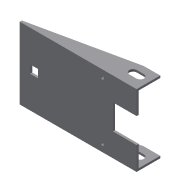
# Autodesk Inventor part: U-profil 100x40 - pod case
Saved by Autodesk Inventor 2015 (Build 190159000, 159)
## iProperties
Created: 2015-01-09
Part Number: U-profil 100x40 - pod case
Material: Všeobecné
Document SubType Name: Modeling
Designer: Michal
Density: 1 g/cm^3
Appearance: Výchozí
Author: Michal
Autodesk Inventor part; units mm, degrees
ref_plane "YZ Plane" through (0, 0, 0) normal (1, 0, 0) x (0, 1, 0)
ref_plane "XZ Plane" through (0, 0, 0) normal (0, 1, 0) x (-1, 0, 0)
ref_plane "XY Plane" through (0, 0, 0) normal (0, 0, 1) x (1, 0, 0)
sketch "Náčrt1" plane through (0, 0, 0) normal (1, 0, 0) x (0, 1, 0)
  line L0 (0, 0) -> (0, -100)
  line L1 (0, -100) -> (33, -100)
  line L2 (33, -100) -> (33, -97)
  line L3 (33, -97) -> (3, -97)
  line L4 (3, -97) -> (3, -3)
  line L5 (3, -3) -> (33, -3)
  line L6 (33, -3) -> (33, 0)
  line L7 (33, 0) -> (0, 0)
  dimension "d0" = 100
  dimension "d1" = 33
  dimension "d2" = 3
  dimension "d3" = 30
  dimension "d4" = 94
  dimension "d5" = 30
  dimension "d6" = 3
  constraints: 16 end point, 4 perpendicular, 2 point on line, 1 vertical
  measures "d0" distance of L0.start L0.end
  measures "d1" distance of L0.end L1.end
  measures "d2" distance of L1.end L2.end
  measures "d3" distance of L2.end L3.end
  measures "d4" distance of L3.end L4.end
  measures "d5" distance of L4.end L5.end
  measures "d6" distance of L5.end L6.end
extrude "Vysunutí1" add sketch "Náčrt1" along normal blind 160
sketch "Náčrt4" plane through (0, 3, -3) normal (0, 1, 0) x (1, 0, 0)
  line L0 (0, 94) -> (0, 0) projected
  line L1 (0, 0) -> (160, 0) projected
  line L2 (160, 94) -> (160, 0) projected
  line L3 (0, 94) -> (160, 94) projected
  line L4 (14.35, 52.65) -> (25.65, 52.65)
  line L5 (25.65, 52.65) -> (25.65, 41.35)
  line L6 (25.65, 41.35) -> (14.35, 41.35)
  line L7 (14.35, 41.35) -> (14.35, 52.65)
  line L8 (0, 97) -> (160, 97) projected
  point P0 (0, -3)
  point P1 (20, 41.35)
  point P2 (14.35, 47)
  dimension "d104" = 11.3
  dimension "d105" = 11.3
  dimension "d106" = 50
  dimension "d107" = 140
  constraints: 8 end point, 2 midpoint, 2 parallel, 1 horizontal, 1 perpendicular
  measures "d104" distance of L5.end L6.end
  measures "d105" distance of L6.end L4.start
  measures "d106" distance from line of L8 point (14.35, 47)
  measures "d107" distance from line of L2 point (20, 41.35)
extrude "Vysunutí4" cut sketch "Náčrt4" against normal through all contours L4 L5 L6 L7
sketch "Náčrt7" plane through (0, 0, -100) normal (0, -1, 0) x (1, 0, 0)
  line L0 (0, 100) -> (0, 0) projected
  line L1 (0, 0) -> (160, 0) projected
  line L2 (160, 100) -> (160, 0) projected
  line L3 (0, 100) -> (160, 100) projected
  circle A0 centre (115, 90) radius 2.25
  circle A1 centre (115, 10) radius 2.25
  dimension "d76" = 4.5
  dimension "d77" = 4.5
  dimension "d78" = 10
  dimension "d79" = 10
  dimension "d80" = 115
  dimension "d81" = 115
  constraints: 2 centre point
  measures "d76" diameter of A0
  measures "d77" diameter of A1
  measures "d78" distance from line of L3 A0.centre
  measures "d79" distance from line of L1 A1.centre
  measures "d80" distance from line of A1.centre L0
  measures "d81" distance from line of L0 A0.centre
extrude "Vysunutí7" cut sketch "Náčrt7" against normal through all contours A0 | A1
sketch "Náčrt8" plane through (0, 0, -100) normal (0, 0, -1) x (-1, 0, 0)
  line L0 (0, 0) -> (0, 33) projected
  line L1 (0, 33) -> (-160, 33) projected
  line L2 (-160, 0) -> (-160, 33) projected
  line L3 (0, 0) -> (-160, 0) projected
  line L4 (0, 3) -> (-160, 3) projected
  line L5 (0, 0) -> (0, 33) projected
  line L6 (0, 3) -> (-140, 33)
  line L7 (0, 33) -> (-160, 33) projected
  line L8 (0, 3) -> (0, 33)
  line L9 (0, 33) -> (-140, 33)
  dimension "d85" = 140
  dimension "d86" = 30
  constraints: 6 end point, 2 point on line, 1 collinear, 1 vertical
  measures "d85" distance from line of L0 L6.end
  measures "d86" distance from line of L6.start L1
extrude "Vysunutí8" cut sketch "Náčrt8" against normal through all contours L6 L1 L0
sketch "Náčrt9" plane through (0, 0, -100) normal (0, -1, 0) x (1, 0, 0)
  circle A0 centre (115, 90) radius 2.25 projected
  circle A1 centre (115, 10) radius 2.25 projected
  line L0 (0, 100) -> (0, 0) projected
  line L1 (0, 0) -> (160, 0) projected
  line L2 (160, 100) -> (160, 0) projected
  line L3 (0, 100) -> (160, 100) projected
  line L4 (130, 67.5) -> (160, 67.5)
  line L5 (160, 67.5) -> (160, 32.5)
  line L6 (160, 32.5) -> (130, 32.5)
  line L7 (130, 32.5) -> (130, 67.5)
  line L8 (160, 100) -> (160, 0) projected
  point P0 (130, 50)
  dimension "d90" = 35
  dimension "d91" = 50
  dimension "d92" = 30
  dimension "d93" = 30
  constraints: 8 end point, 2 parallel, 1 collinear, 1 horizontal, 1 midpoint, 1 perpendicular
  measures "d90" distance of L6.end L4.start
  measures "d91" distance from line of L3 point (130, 50)
  measures "d92" distance of L4.start L4.end
  measures "d93" distance between parallel lines of L2 L7
extrude "Vysunutí9" cut sketch "Náčrt9" against normal through all contours L2 L6 L7 L4
sketch "Náčrt10" plane through (160, 0, 0) normal (1, 0, 0) x (0, 0, -1)
  line L0 (67.5, 3) -> (67.5, 0) projected
  line L1 (67.5, 0) -> (100, 0) projected
  line L2 (100, 0) -> (100, 33) projected
  line L3 (100, 33) -> (97, 33) projected
  line L4 (97, 33) -> (97, 3) projected
  line L5 (97, 3) -> (67.5, 3) projected
  line L6 (32.5, 0) -> (32.5, 3) projected
  line L7 (32.5, 3) -> (3, 3) projected
  line L8 (3, 3) -> (3, 33) projected
  line L9 (3, 33) -> (0, 33) projected
  line L10 (0, 33) -> (0, 0) projected
  line L11 (0, 0) -> (32.5, 0) projected
extrude "Vysunutí10" add sketch "Náčrt10" along normal blind 3
sketch "Náčrt11" plane through (0, 0, 0) normal (0, 0, 1) x (1, 0, 0)
  line L0 (140, 33) -> (0, 3) projected
  line L1 (0, 3) -> (0, 0) projected
  line L2 (0, 0) -> (163, 0) projected
  line L3 (163, 33) -> (163, 0) projected
  line L4 (140, 33) -> (163, 33) projected
  arc A0 (150, 12.75) -> (150, 23.25) centre (150, 18) ccw
  arc A1 (140, 23.25) -> (140, 12.75) centre (140, 18) ccw
  line L5 (150, 12.75) -> (140, 12.75)
  line L6 (140, 23.25) -> (150, 23.25)
  dimension "d98" = 10.5
  dimension "d99" = 10.5
  dimension "d100" = 10
  dimension "d101" = 13
  dimension "d108" = 15
  constraints: 4 end point, 4 point on circle, 2 centre point, 2 tangent, 1 parallel
  measures "d98" diameter of A0
  measures "d99" diameter of A1
  measures "d100" distance of A1.centre A0.centre
  measures "d101" distance from line of L3 A0.centre
  measures "d108" distance from line of L4 A0.centre
extrude "Vysunutí11" cut sketch "Náčrt11" against normal through all contours L5 A1 L6 A0
